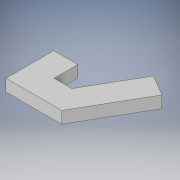
# Autodesk Inventor part: S claw half
Saved by Autodesk Inventor 2018.2 (Build 222227000, 227)
## iProperties
Created: 2018-01-13
Part Number: S claw half
Material: Generic
Document SubType Name: Modeling
Designer: jahu2
Density: 1 g/cm^3
Appearance: Default
Author: jahu2
Autodesk Inventor part; units mm, degrees
ref_plane "YZ Plane" through (0, 0, 0) normal (1, 0, 0) x (0, 1, 0)
ref_plane "XZ Plane" through (0, 0, 0) normal (0, 1, 0) x (-1, 0, 0)
ref_plane "XY Plane" through (0, 0, 0) normal (0, 0, 1) x (1, 0, 0)
sketch "Sketch5" plane through (0, 0, 0) normal (0, 1, 0) x (-1, 0, 0)
  line L0 (0, 0) -> (0, 38.1)
  line L1 (0, 38.1) -> (-38.1, 38.1)
  line L2 (-38.1, 38.1) -> (-101.6, -71.8852)
  line L3 (51.1953, 0) -> (51.1953, 89.2953)
  line L4 (51.1953, 89.2953) -> (-67.6576, 89.2953)
  line L5 (-67.6576, 89.2953) -> (-145.9365, -46.2876)
  line L6 (-101.6, -71.8852) -> (-145.9365, -46.2876)
  line L7 (0, 0) -> (0, -12.7)
  line L8 (51.1953, 0) -> (51.1953, -12.7)
  line L9 (51.1953, 0) -> (63.8953, 0) construction
  line L10 (51.1953, -12.7) -> (0, -12.7)
  dimension "d33" = 38.1
  dimension "d34" = 38.1
  dimension "d35" = 127
  dimension "d36" = 120
  dimension "d37" = 51.1953
  dimension "d38" = 12.7
  dimension "d39" = 12.7
  dimension "d40" = 90
  constraints: 22 end point, 3 perpendicular, 3 vertical, 2 horizontal, 2 other
  measures "d33" distance of L0.start L0.end
  measures "d34" distance of L0.end L1.end
  measures "d35" distance of L1.end L2.end
  measures "d36" angle of L2 L1
  measures "d37" distance between parallel lines of L0 L3
  measures "d38" distance of L0.start L7.end
  measures "d39" distance of L3.start L8.end
  measures "d40" angle of L8 L9
extrude "Extrusion4" add sketch "Sketch5" along normal blind 25.4
body "Solid4"
